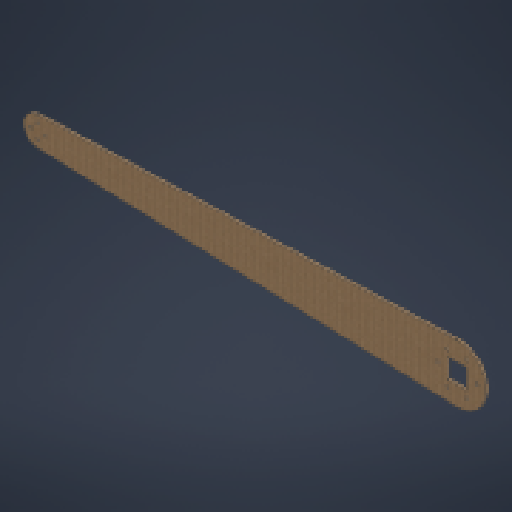
# Autodesk Inventor part: MainArm
Saved by Autodesk Inventor 2024.1 (Build 281209000, 209)
## iProperties
Created: 2023-10-16
Part Number: MainArm
Material: MDF Medium Density Fiberboard
Document SubType Name: Modeling
Designer: Brandon
Density: 0.8 g/cm^3
Appearance: Cardboard - Corrugated
Author: Brandon
Autodesk Inventor part; units mm, degrees
ref_plane "YZ Plane" through (0, 0, 0) normal (1, 0, 0) x (0, 1, 0)
ref_plane "XZ Plane" through (0, 0, 0) normal (0, 1, 0) x (-1, 0, 0)
ref_plane "XY Plane" through (0, 0, 0) normal (0, 0, 1) x (1, 0, 0)
sketch "Sketch1" plane through (0, 0, 0) normal (0, 0, 1) x (1, 0, 0)
  circle A0 centre (0, 0) radius 31.75 projected
  circle A1 centre (25.4, 0) radius 2.1 projected
  circle A2 centre (-25.4, 0) radius 2.1 projected
  circle A3 centre (12.7, -21.997) radius 2.1 projected
  circle A4 centre (-12.7, -21.997) radius 2.1 projected
  line L0 (12.7, -12.7) -> (12.7, 12.7) projected
  line L1 (-12.7, -12.7) -> (12.7, -12.7) projected
  line L2 (-12.7, 12.7) -> (-12.7, -12.7) projected
  line L3 (12.7, 12.7) -> (-12.7, 12.7) projected
  circle A5 centre (12.7, 21.997) radius 2.1 projected
  circle A6 centre (-12.7, 21.997) radius 2.1 projected
  circle A7 centre (0, 0) radius 38.1
  line L4 (0, 0) -> (-550, 0)
  circle A8 centre (-550, 0) radius 19.05
  circle A9 centre (-540.475, 0) radius 2
  circle A10 centre (-550, 9.525) radius 2
  circle A11 centre (-559.525, 0) radius 2
  circle A12 centre (-550, -9.525) radius 2
  line L5 (-1.3196, 38.0771) -> (-550.6598, 19.0386)
  line L6 (-1.3196, -38.0771) -> (-550.6598, -19.0386)
  circle A13 centre (12.7, 21.997) radius 2
  circle A14 centre (-12.7, 21.997) radius 2
  circle A15 centre (25.4, 0) radius 2
  circle A16 centre (-25.4, 0) radius 2
  circle A17 centre (12.7, -21.997) radius 2
  circle A18 centre (-12.7, -21.997) radius 2
  dimension "d0" = 76.2
  dimension "d1" = 550
  dimension "d2" = 38.1
  dimension "d3" = 4
  dimension "d4" = 9.525
  dimension "d7" = 360
  dimension "d9" = 4
  dimension "d10" = 4
  dimension "d11" = 4
  dimension "d12" = 4
  dimension "d13" = 4
  dimension "d14" = 4
  constraints: 12 centre point, 8 coincident, 6 end point, 4 point on circle, 4 tangent, 1 horizontal, 1 point on line, 9 other
  measures "d0" diameter of A7
  measures "d1" distance of L4.start L4.end
  measures "d2" diameter of A8
  measures "d3" diameter of A9
  measures "d4" distance of L4.end A9.centre
  measures "d9" diameter of A13
  measures "d10" diameter of A14
  measures "d11" diameter of A15
  measures "d12" diameter of A16
  measures "d13" diameter of A17
  measures "d14" diameter of A18
extrude "Extrusion1" add sketch "Sketch1" along normal blind 3.175 contours A0 | A7 | A7 L4 A8 L5 | L6 A8 L4 A7 | A8
body "Solid1"
